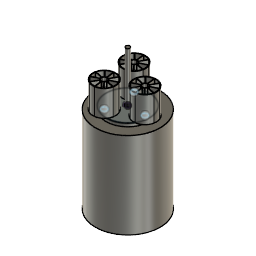
Peristaltic_Pump (Autodesk Fusion 360 design; units mm, degrees)
Autodesk Fusion 360 part; units mm, degrees
sketch "Sketch1" plane through (0, 0, 0) normal (0, 0, 1) x (1, 0, 0)
  circle A0 centre (0, 0) radius 15
  dimension "d1" = 30
  constraint coincident A0.centre origin
  measures "d1" diameter of A0
extrude "Extrude1" add sketch "Sketch1" along normal blind 40 makes body 1
sketch "Sketch2" plane through (0, 0, 40) normal (0, 0, 1) x (-1, 0, 0)
  circle A0 centre (0, 0) radius 15
  circle A1 centre (0, 0) radius 1
  dimension "d4" = 2
  constraint coincident A0.centre A1.centre
  measures "d4" diameter of A1
extrude "Extrude2" add sketch "Sketch2" along normal blind 25 contours A1 bodies 1
copy_body "Body->Comp1" bodies 1 removing the originals makes body 2 in component "MOTOR"
sketch "Sketch1 (2)" plane through (0, 0, 0) normal (0, 0, 1) x (1, 0, 0) in component "disc v3"
  circle A0 centre (0, 0) radius 10
  circle A1 centre (0, 0) radius 1
  circle A2 centre (0, 8) radius 1.25
  circle A3 centre (-6.9282, -4) radius 1.25
  circle A4 centre (6.9282, -4) radius 1.25
  dimension "d1_1" = 20
  dimension "d2_1" = 2
  dimension "d5_1" = 2.5
  constraint coincident A0.centre A1.centre
  measures "d1_1" diameter of A0
  measures "d2_1" diameter of A1
  measures "d5_1" diameter of A2
extrude "Extrude1'" add sketch "Sketch1 (2)" against normal blind 1.5 separate body contours A0 | A2 | A3 | A4 makes body 3 in component "disc v3"
extrude "Extrude2'" add sketch "Sketch1 (2)" along normal blind 10 contours A2 | A3 | A4 bodies 3 in component "disc v3"
sketch "Sketch1 (3)" plane through (0, 0, 0) normal (0, 0, 1) x (1, 0, 0) in component "roller_1"
  circle A0 centre (0, 0) radius 5
  circle A1 centre (0, 0) radius 1.5
  line L0 (0, 1.5) -> (0, 5)
  line L1 (-0.0675, 1.4985) -> (-0.2252, 5)
  line L2 (-0.9354, 1.1726) -> (-3.1211, 3.9127)
  line L3 (-0.8817, 1.2135) -> (-2.9389, 4.0451)
  line L4 (-1.446, 0.3989) -> (-4.8249, 1.331)
  line L5 (-1.4266, 0.4635) -> (-4.7553, 1.5451)
  line L6 (-1.4043, -0.5272) -> (-4.6857, -1.7592)
  line L7 (-1.4266, -0.4635) -> (-4.7553, -1.5451)
  line L8 (-0.8262, -1.252) -> (-2.7568, -4.1774)
  line L9 (-0.8817, -1.2135) -> (-2.9389, -4.0451)
  line L10 (0.0675, -1.4985) -> (0.2252, -5)
  line L11 (0, -1.5) -> (0, -5)
  line L12 (0.9354, -1.1726) -> (3.1211, -3.9127)
  line L13 (0.8817, -1.2135) -> (2.9389, -4.0451)
  line L14 (1.446, -0.3989) -> (4.8249, -1.331)
  line L15 (1.4266, -0.4635) -> (4.7553, -1.5451)
  line L16 (1.4043, 0.5272) -> (4.6857, 1.7592)
  line L17 (1.4266, 0.4635) -> (4.7553, 1.5451)
  line L18 (0.8262, 1.252) -> (2.7568, 4.1774)
  line L19 (0.8817, 1.2135) -> (2.9389, 4.0451)
  circle A2 centre (0, 0) radius 5.263
  circle A3 centre (0, 0) radius 1.25
  dimension "d1_2" = 10
  dimension "d2_2" = 3
  dimension "d7_1" = 2.5
  constraint coincident A0.centre A1.centre
  constraint coincident A0 L0.end
  constraint vertical L0
  constraint coincident A1 L3.start
  constraint coincident A1 L2.start
  constraint coincident A1 L1.start
  constraint coincident A1 L18.start
  constraint coincident A1 L19.start
  constraint coincident A1 L16.start
  constraint coincident A1 L17.start
  constraint coincident A1 L14.start
  constraint coincident A1 L15.start
  constraint coincident A1 L12.start
  constraint coincident A1 L13.start
  constraint coincident A1 L10.start
  constraint coincident A1 L11.start
  constraint coincident A1 L8.start
  constraint coincident A1 L9.start
  constraint coincident A1 L6.start
  constraint coincident A1 L7.start
  constraint coincident A1 L4.start
  constraint coincident A1 L5.start
  constraint coincident A1 L0.start
  measures "d1_2" diameter of A0
  measures "d2_2" diameter of A1
  measures "d7_1" diameter of A3
extrude "Extrude1''" add sketch "Sketch1 (3)" along normal blind 12 separate body contours A0 A1 L16 L17 | A0 A1 L14 L15 | A1 | A0 A1 L18 L19 | A0 A1 L12 L13 | A0 A1 L0 L1 | A0 A1 L10 L11 | A0 A1 L2 L3 | A0 A1 L8 L9 | A0 A1 L4 L5 | A0 A1 L6 L7 | A2 makes body 4 in component "roller_1"
sketch "Sketch1 (4)" plane through (0, 0, 0) normal (0, 0, 1) x (1, 0, 0) in component "roller_2"
  circle A0 centre (0, 0) radius 5
  circle A1 centre (0, 0) radius 1.5
  line L0 (0, 1.5) -> (0, 5)
  line L1 (-0.0675, 1.4985) -> (-0.2252, 5)
  line L2 (-0.9354, 1.1726) -> (-3.1211, 3.9127)
  line L3 (-0.8817, 1.2135) -> (-2.9389, 4.0451)
  line L4 (-1.446, 0.3989) -> (-4.8249, 1.331)
  line L5 (-1.4266, 0.4635) -> (-4.7553, 1.5451)
  line L6 (-1.4043, -0.5272) -> (-4.6857, -1.7592)
  line L7 (-1.4266, -0.4635) -> (-4.7553, -1.5451)
  line L8 (-0.8262, -1.252) -> (-2.7568, -4.1774)
  line L9 (-0.8817, -1.2135) -> (-2.9389, -4.0451)
  line L10 (0.0675, -1.4985) -> (0.2252, -5)
  line L11 (0, -1.5) -> (0, -5)
  line L12 (0.9354, -1.1726) -> (3.1211, -3.9127)
  line L13 (0.8817, -1.2135) -> (2.9389, -4.0451)
  line L14 (1.446, -0.3989) -> (4.8249, -1.331)
  line L15 (1.4266, -0.4635) -> (4.7553, -1.5451)
  line L16 (1.4043, 0.5272) -> (4.6857, 1.7592)
  line L17 (1.4266, 0.4635) -> (4.7553, 1.5451)
  line L18 (0.8262, 1.252) -> (2.7568, 4.1774)
  line L19 (0.8817, 1.2135) -> (2.9389, 4.0451)
  circle A2 centre (0, 0) radius 5.263
  circle A3 centre (0, 0) radius 1.25
  dimension "d1_3" = 10
  dimension "d2_3" = 3
  dimension "d7_2" = 2.5
  constraint coincident A0.centre A1.centre
  constraint coincident A0 L0.end
  constraint vertical L0
  constraint coincident A1 L3.start
  constraint coincident A1 L2.start
  constraint coincident A1 L1.start
  constraint coincident A1 L18.start
  constraint coincident A1 L19.start
  constraint coincident A1 L16.start
  constraint coincident A1 L17.start
  constraint coincident A1 L14.start
  constraint coincident A1 L15.start
  constraint coincident A1 L12.start
  constraint coincident A1 L13.start
  constraint coincident A1 L10.start
  constraint coincident A1 L11.start
  constraint coincident A1 L8.start
  constraint coincident A1 L9.start
  constraint coincident A1 L6.start
  constraint coincident A1 L7.start
  constraint coincident A1 L4.start
  constraint coincident A1 L5.start
  constraint coincident A1 L0.start
  measures "d1_3" diameter of A0
  measures "d2_3" diameter of A1
  measures "d7_2" diameter of A3
extrude "Extrude1'''" add sketch "Sketch1 (4)" along normal blind 12 separate body contours A0 A1 L16 L17 | A0 A1 L14 L15 | A1 | A0 A1 L18 L19 | A0 A1 L12 L13 | A0 A1 L0 L1 | A0 A1 L10 L11 | A0 A1 L2 L3 | A0 A1 L8 L9 | A0 A1 L4 L5 | A0 A1 L6 L7 | A2 makes body 5 in component "roller_2"
sketch "Sketch1 (5)" plane through (0, 0, 0) normal (0, 0, 1) x (1, 0, 0) in component "roller_3"
  circle A0 centre (0, 0) radius 5
  circle A1 centre (0, 0) radius 1.5
  line L0 (0, 1.5) -> (0, 5)
  line L1 (-0.0675, 1.4985) -> (-0.2252, 5)
  line L2 (-0.9354, 1.1726) -> (-3.1211, 3.9127)
  line L3 (-0.8817, 1.2135) -> (-2.9389, 4.0451)
  line L4 (-1.446, 0.3989) -> (-4.8249, 1.331)
  line L5 (-1.4266, 0.4635) -> (-4.7553, 1.5451)
  line L6 (-1.4043, -0.5272) -> (-4.6857, -1.7592)
  line L7 (-1.4266, -0.4635) -> (-4.7553, -1.5451)
  line L8 (-0.8262, -1.252) -> (-2.7568, -4.1774)
  line L9 (-0.8817, -1.2135) -> (-2.9389, -4.0451)
  line L10 (0.0675, -1.4985) -> (0.2252, -5)
  line L11 (0, -1.5) -> (0, -5)
  line L12 (0.9354, -1.1726) -> (3.1211, -3.9127)
  line L13 (0.8817, -1.2135) -> (2.9389, -4.0451)
  line L14 (1.446, -0.3989) -> (4.8249, -1.331)
  line L15 (1.4266, -0.4635) -> (4.7553, -1.5451)
  line L16 (1.4043, 0.5272) -> (4.6857, 1.7592)
  line L17 (1.4266, 0.4635) -> (4.7553, 1.5451)
  line L18 (0.8262, 1.252) -> (2.7568, 4.1774)
  line L19 (0.8817, 1.2135) -> (2.9389, 4.0451)
  circle A2 centre (0, 0) radius 5.263
  circle A3 centre (0, 0) radius 1.25
  dimension "d1_4" = 10
  dimension "d2_4" = 3
  dimension "d7_3" = 2.5
  constraint coincident A0.centre A1.centre
  constraint coincident A0 L0.end
  constraint vertical L0
  constraint coincident A1 L3.start
  constraint coincident A1 L2.start
  constraint coincident A1 L1.start
  constraint coincident A1 L18.start
  constraint coincident A1 L19.start
  constraint coincident A1 L16.start
  constraint coincident A1 L17.start
  constraint coincident A1 L14.start
  constraint coincident A1 L15.start
  constraint coincident A1 L12.start
  constraint coincident A1 L13.start
  constraint coincident A1 L10.start
  constraint coincident A1 L11.start
  constraint coincident A1 L8.start
  constraint coincident A1 L9.start
  constraint coincident A1 L6.start
  constraint coincident A1 L7.start
  constraint coincident A1 L4.start
  constraint coincident A1 L5.start
  constraint coincident A1 L0.start
  measures "d1_4" diameter of A0
  measures "d2_4" diameter of A1
  measures "d7_3" diameter of A3
extrude "Extrude1''''" add sketch "Sketch1 (5)" along normal blind 12 separate body contours A0 A1 L16 L17 | A0 A1 L14 L15 | A1 | A0 A1 L18 L19 | A0 A1 L12 L13 | A0 A1 L0 L1 | A0 A1 L10 L11 | A0 A1 L2 L3 | A0 A1 L8 L9 | A0 A1 L4 L5 | A0 A1 L6 L7 | A2 makes body 6 in component "roller_3"
component "MOTOR" placed x (1, 0, 0) y (0, 1, 0) z (0, 0, 1) at (0, 0, 0)
component "disc v3" placed x (-0.866025, 0.5, 0) y (-0.5, -0.866025, 0) z (0, 0, 1) at (0, 0, 41.5)
component "roller_1" placed x (0.866025, -0.5, 0) y (0.5, 0.866025, 0) z (0, 0, 1) at (-4, 6.9282, 41.5)
component "roller_2" placed x (0.866025, -0.5, 0) y (0.5, 0.866025, 0) z (0, 0, 1) at (-4, -6.9282, 41.5)
component "roller_3" placed x (0.866025, -0.5, 0) y (0.5, 0.866025, 0) z (0, 0, 1) at (8, 0, 41.5)
